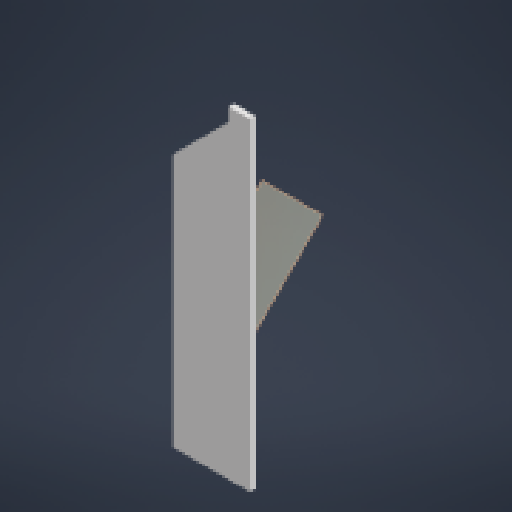
# Autodesk Inventor part: BokPrawy
Saved by Autodesk Inventor 2023 (Build 270158000, 158)
## iProperties
Created: 2023-03-15
Part Number: BokPrawy
Material: Generic
Document SubType Name: Modeling
Designer: Michał
Density: 1 g/cm^3
Appearance: Default
Author: Michał
Autodesk Inventor part; units mm, degrees
ref_plane "YZ Plane" through (0, 0, 0) normal (1, 0, 0) x (0, 1, 0)
ref_plane "XZ Plane" through (0, 0, 0) normal (0, 1, 0) x (-1, 0, 0)
ref_plane "XY Plane" through (0, 0, 0) normal (0, 0, 1) x (1, 0, 0)
sketch "Sketch1" plane through (0, 0, 0) normal (0, 0, 1) x (1, 0, 0)
  line L0 (17.2892, -53.3685) -> (9.2892, -53.3685) projected
  line L1 (-10.7108, -53.3685) -> (9.2892, -53.3685) projected
  line L2 (9.2892, 58.6315) -> (-10.7108, 38.6315) projected
  line L3 (17.2892, -53.3685) -> (17.2892, -49.7758) projected
  line L4 (17.2892, -46.9611) -> (17.2892, 27.2242) projected
  line L5 (17.2892, 30.0389) -> (17.2892, 41.6315) projected
  line L6 (17.2892, 41.6315) -> (17.2892, 51.5315) projected
  line L7 (17.2892, 63.6315) -> (17.2892, 56.6315) projected
  line L8 (9.2892, 63.6315) -> (17.2892, 63.6315) construction
  line L9 (17.2892, 63.6315) -> (9.5892, 63.6315)
  line L10 (9.5892, 63.6315) -> (9.5892, 59.3458)
  line L11 (9.2892, 58.6315) -> (9.2963, 58.6387)
  line L12 (9.2892, 60.6315) -> (9.2892, 63.6315) construction
  arc A0 (9.2963, 58.6387) -> (9.5892, 59.3458) centre (8.5892, 59.3458) ccw
  line L13 (17.2892, 27.2242) -> (17.2892, 30.0389)
  line L14 (17.2892, 51.5315) -> (17.2892, 56.6315)
  line L15 (17.2892, -49.7758) -> (17.2892, -46.9611)
  line L16 (-10.7108, -53.3685) -> (-12.7108, -53.3685)
  line L17 (-12.7108, -53.3685) -> (-12.7108, 36.6315)
  line L18 (-12.7108, 36.6315) -> (-10.7108, 38.6315)
  point P0 (0, 0)
  dimension "d2" = 0.3
  dimension "d3" = 1
  dimension "d19" = 30
  constraints: 18 end point, 3 collinear, 2 point on circle, 2 tangent, 2 vertical, 1 centre point, 1 horizontal, 1 perpendicular, 1 point on line
  measures "d2" distance between parallel lines of L12 L10
  measures "d3" radius of A0
  measures "d19" distance between parallel lines of L4 L17
extrude "Extrusion1" add sketch "Sketch1" along normal blind 3
ref_plane "Work Plane2" through (4.04, -8.0435, 0.345) normal (0, 0.7071, 0.7071) x (1, 0, 0)
sketch "Sketch3" plane through (4.04, -8.0435, 0.345) normal (0, 0.7071, 0.7071) x (1, 0, 0)
  line L0 (-4, 22) -> (-4, 0) construction
  line L1 (4, 22) -> (-4, 22) construction
  line L2 (4, 0) -> (4, 22) construction
  line L3 (-4, 0) -> (4, 0) construction
  line L4 (-5.5, 23.5) -> (-5.5, -1.5)
  line L5 (-5.5, 23.5) -> (5.5, 23.5)
  line L6 (5.5, 23.5) -> (5.5, -1.5)
  line L7 (5.5, -1.5) -> (-5.5, -1.5)
  point P0 (-4.04, 5.9315)
  dimension "d6" = 1.5
  dimension "d7" = 1.5
  dimension "d8" = 1.5
  dimension "d9" = 1.5
  constraints: 8 end point, 2 parallel, 2 perpendicular
  measures "d6" distance between parallel lines of L4 L0
  measures "d7" distance between parallel lines of L5 L1
  measures "d8" distance between parallel lines of L6 L2
  measures "d9" distance between parallel lines of L7 L3
extrude "Extrusion2" cut sketch "Sketch3" along normal through all
sketch "Sketch4" plane through (0, 0, 3) normal (0, 0, 1) x (1, 0, 0)
  circle A0 centre (-5.7108, -43.3685) radius 2.25 projected
  circle A1 centre (4.2892, -43.3685) radius 2.25 projected
  circle A2 centre (-5.7108, 36.6315) radius 2.25 projected
  circle A3 centre (4.2892, 36.6315) radius 2.25 projected
  point P0 (0, 0)
  constraints: 4 coincident
hole "Hole1" at (-5.7108, -43.3685, 3) at (4.2892, -43.3685, 3) at (-5.7108, 36.6315, 3) at (4.2892, 36.6315, 3) direction (0, 0, -1) diameter 3.4 end through all countersink diameter 6.3 countersink angle 90 clearance for "Countersunk Flat Head Screw ISO 2009/7046" size "M3" standard "ISO"
equation "\"d7\" = d6"
equation "\"d8\" = d6"
equation "\"d9\" = d6"
body "Solid1"
